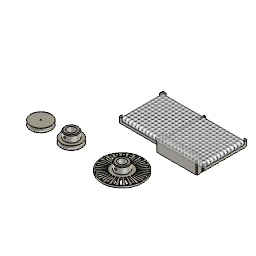
test_parts_v1 (Autodesk Fusion 360 design; units mm, degrees)
Autodesk Fusion 360 part; units mm, degrees
sketch "スケッチ1" plane through (0, 0, 0) normal (0, 0, 1) x (1, 0, 0)
  circle A0 centre (0, 0) radius 30
  circle A1 centre (0, 0) radius 6
  circle A2 centre (0, 0) radius 28.5
  circle A3 centre (0, 0) radius 10
  line L0 (0, -10) -> (0, -28.5)
  line L1 (1.3053, -9.9144) -> (3.72, -28.2562)
  line L2 (2.5882, -9.6593) -> (7.3763, -27.5289)
  line L3 (3.8268, -9.2388) -> (10.9065, -26.3306)
  line L4 (5, -8.6603) -> (14.25, -24.6817)
  line L5 (6.0876, -7.9335) -> (17.3497, -22.6106)
  line L6 (7.0711, -7.0711) -> (20.1525, -20.1525)
  line L7 (7.9335, -6.0876) -> (22.6106, -17.3497)
  line L8 (8.6603, -5) -> (24.6817, -14.25)
  line L9 (9.2388, -3.8268) -> (26.3306, -10.9065)
  line L10 (9.6593, -2.5882) -> (27.5289, -7.3763)
  line L11 (9.9144, -1.3053) -> (28.2562, -3.72)
  line L12 (10, 0) -> (28.5, 0)
  line L13 (9.9144, 1.3053) -> (28.2562, 3.72)
  line L14 (9.6593, 2.5882) -> (27.5289, 7.3763)
  line L15 (9.2388, 3.8268) -> (26.3306, 10.9065)
  line L16 (8.6603, 5) -> (24.6817, 14.25)
  line L17 (7.9335, 6.0876) -> (22.6106, 17.3497)
  line L18 (7.0711, 7.0711) -> (20.1525, 20.1525)
  line L19 (6.0876, 7.9335) -> (17.3497, 22.6106)
  line L20 (5, 8.6603) -> (14.25, 24.6817)
  line L21 (3.8268, 9.2388) -> (10.9065, 26.3306)
  line L22 (2.5882, 9.6593) -> (7.3763, 27.5289)
  line L23 (1.3053, 9.9144) -> (3.72, 28.2562)
  line L24 (0, 10) -> (0, 28.5)
  line L25 (-1.3053, 9.9144) -> (-3.72, 28.2562)
  line L26 (-2.5882, 9.6593) -> (-7.3763, 27.5289)
  line L27 (-3.8268, 9.2388) -> (-10.9065, 26.3306)
  line L28 (-5, 8.6603) -> (-14.25, 24.6817)
  line L29 (-6.0876, 7.9335) -> (-17.3497, 22.6106)
  line L30 (-7.0711, 7.0711) -> (-20.1525, 20.1525)
  line L31 (-7.9335, 6.0876) -> (-22.6106, 17.3497)
  line L32 (-8.6603, 5) -> (-24.6817, 14.25)
  line L33 (-9.2388, 3.8268) -> (-26.3306, 10.9065)
  line L34 (-9.6593, 2.5882) -> (-27.5289, 7.3763)
  line L35 (-9.9144, 1.3053) -> (-28.2562, 3.72)
  line L36 (-10, 0) -> (-28.5, 0)
  line L37 (-9.9144, -1.3053) -> (-28.2562, -3.72)
  line L38 (-9.6593, -2.5882) -> (-27.5289, -7.3763)
  line L39 (-9.2388, -3.8268) -> (-26.3306, -10.9065)
  line L40 (-8.6603, -5) -> (-24.6817, -14.25)
  line L41 (-7.9335, -6.0876) -> (-22.6106, -17.3497)
  line L42 (-7.0711, -7.0711) -> (-20.1525, -20.1525)
  line L43 (-6.0876, -7.9335) -> (-17.3497, -22.6106)
  line L44 (-5, -8.6603) -> (-14.25, -24.6817)
  line L45 (-3.8268, -9.2388) -> (-10.9065, -26.3306)
  line L46 (-2.5882, -9.6593) -> (-7.3763, -27.5289)
  line L47 (-1.3053, -9.9144) -> (-3.72, -28.2562)
  dimension "d1" = 60
  dimension "d2" = 12
  dimension "d3" = 57
  dimension "d5" = 360
  constraint coincident A0.centre A1.centre
  constraint concentric A0 A2
  constraint concentric A2 A3
  constraint coincident A2 L0.end
  constraint coincident A3 L0.start
  measures "d1" diameter of A0
  measures "d2" diameter of A1
  measures "d3" diameter of A2
extrude "押し出し1" add sketch "スケッチ1" along normal blind 3 contours A0 | A2 A3 L12 L13 | A2 A3 L10 L11 | A3 | A2 A3 L14 L15 | A2 A3 L8 L9 | A2 A3 L16 L17 | A2 A3 L6 L7 | A2 A3 L18 L19 | A2 A3 L4 L5 | A2 A3 L20 L21 | A2 A3 L2 L3 | A2 A3 L22 L23 | A2 A3 L0 L1 | A2 A3 L24 L25 | A2 A3 L46 L47 | A2 A3 L26 L27 | A2 A3 L44 L45 | A2 A3 L28 L29 | A2 A3 L42 L43 | A2 A3 L30 L31 | A2 A3 L40 L41 | A2 A3 L32 L33 | A2 A3 L38 L39 | A2 A3 L34 L35 | A2 A3 L36 L37 makes body 1
sketch "スケッチ2" plane through (0, 0, 0) normal (0, 0, 1) x (1, 0, 0)
  circle A0 centre (0, 0) radius 15
  circle A1 centre (0, 0) radius 6
  circle A2 centre (0, 0) radius 6
  constraint coincident A0.centre A1.centre
  constraint concentric A0 A2
extrude "押し出し2" add sketch "スケッチ2" along normal blind 3 bodies 1
sketch "スケッチ3" plane through (0, 0, 3) normal (0, 0, 1) x (-1, 0, 0)
  line L0 (3.8823, -14.4889) -> (7.3763, -27.5289)
  arc A0 (3.72, -28.2562) -> (7.3763, -27.5289) centre (0, 0) ccw
  line L1 (3.72, -28.2562) -> (1.9579, -14.8717)
  arc A1 (1.9579, -14.8717) -> (3.8823, -14.4889) centre (0, 0) ccw
  arc A2 (5.7403, -13.8582) -> (7.5, -12.9904) centre (0, 0) ccw
  line L2 (7.5, -12.9904) -> (14.25, -24.6817)
  arc A3 (10.9065, -26.3306) -> (14.25, -24.6817) centre (0, 0) ccw
  line L3 (10.9065, -26.3306) -> (5.7403, -13.8582)
  line L4 (0, -15) -> (0, -28.5)
  arc A4 (-3.72, -28.2562) -> (0, -28.5) centre (0, 0) ccw
  line L5 (-3.72, -28.2562) -> (-1.9579, -14.8717)
  arc A5 (-1.9579, -14.8717) -> (0, -15) centre (0, 0) ccw
  arc A6 (9.1314, -11.9003) -> (10.6066, -10.6066) centre (0, 0) ccw
  line L6 (10.6066, -10.6066) -> (20.1525, -20.1525)
  arc A7 (17.3497, -22.6106) -> (20.1525, -20.1525) centre (0, 0) ccw
  line L7 (17.3497, -22.6106) -> (9.1314, -11.9003)
  line L8 (-3.8823, -14.4889) -> (-7.3763, -27.5289)
  arc A8 (-10.9065, -26.3306) -> (-7.3763, -27.5289) centre (0, 0) ccw
  line L9 (-10.9065, -26.3306) -> (-5.7403, -13.8582)
  arc A9 (-5.7403, -13.8582) -> (-3.8823, -14.4889) centre (0, 0) ccw
  arc A10 (11.9003, -9.1314) -> (12.9904, -7.5) centre (0, 0) ccw
  line L10 (12.9904, -7.5) -> (24.6817, -14.25)
  arc A11 (22.6106, -17.3497) -> (24.6817, -14.25) centre (0, 0) ccw
  line L11 (22.6106, -17.3497) -> (11.9003, -9.1314)
  line L12 (-7.5, -12.9904) -> (-14.25, -24.6817)
  arc A12 (-17.3497, -22.6106) -> (-14.25, -24.6817) centre (0, 0) ccw
  line L13 (-17.3497, -22.6106) -> (-9.1314, -11.9003)
  arc A13 (-9.1314, -11.9003) -> (-7.5, -12.9904) centre (0, 0) ccw
  arc A14 (13.8582, -5.7403) -> (14.4889, -3.8823) centre (0, 0) ccw
  line L14 (14.4889, -3.8823) -> (27.5289, -7.3763)
  arc A15 (26.3306, -10.9065) -> (27.5289, -7.3763) centre (0, 0) ccw
  line L15 (26.3306, -10.9065) -> (13.8582, -5.7403)
  line L16 (-10.6066, -10.6066) -> (-20.1525, -20.1525)
  arc A16 (-22.6106, -17.3497) -> (-20.1525, -20.1525) centre (0, 0) ccw
  line L17 (-22.6106, -17.3497) -> (-11.9003, -9.1314)
  arc A17 (-11.9003, -9.1314) -> (-10.6066, -10.6066) centre (0, 0) ccw
  arc A18 (14.8717, -1.9579) -> (15, 0) centre (0, 0) ccw
  line L18 (15, 0) -> (28.5, 0)
  arc A19 (28.2562, -3.72) -> (28.5, 0) centre (0, 0) ccw
  line L19 (28.2562, -3.72) -> (14.8717, -1.9579)
  line L20 (-12.9904, -7.5) -> (-24.6817, -14.25)
  arc A20 (-26.3306, -10.9065) -> (-24.6817, -14.25) centre (0, 0) ccw
  line L21 (-26.3306, -10.9065) -> (-13.8582, -5.7403)
  arc A21 (-13.8582, -5.7403) -> (-12.9904, -7.5) centre (0, 0) ccw
  arc A22 (14.8717, 1.9579) -> (14.4889, 3.8823) centre (0, 0) ccw
  line L22 (14.4889, 3.8823) -> (27.5289, 7.3763)
  arc A23 (28.2562, 3.72) -> (27.5289, 7.3763) centre (0, 0) ccw
  line L23 (28.2562, 3.72) -> (14.8717, 1.9579)
  line L24 (-14.4889, -3.8823) -> (-27.5289, -7.3763)
  arc A24 (-28.2562, -3.72) -> (-27.5289, -7.3763) centre (0, 0) ccw
  line L25 (-28.2562, -3.72) -> (-14.8717, -1.9579)
  arc A25 (-14.8717, -1.9579) -> (-14.4889, -3.8823) centre (0, 0) ccw
  arc A26 (13.8582, 5.7403) -> (12.9904, 7.5) centre (0, 0) ccw
  line L26 (12.9904, 7.5) -> (24.6817, 14.25)
  arc A27 (26.3306, 10.9065) -> (24.6817, 14.25) centre (0, 0) ccw
  line L27 (26.3306, 10.9065) -> (13.8582, 5.7403)
  line L28 (-15, 0) -> (-28.5, 0)
  arc A28 (-28.2562, 3.72) -> (-28.5, 0) centre (0, 0) ccw
  line L29 (-28.2562, 3.72) -> (-14.8717, 1.9579)
  arc A29 (-14.8717, 1.9579) -> (-15, 0) centre (0, 0) ccw
  arc A30 (11.9003, 9.1314) -> (10.6066, 10.6066) centre (0, 0) ccw
  line L30 (10.6066, 10.6066) -> (20.1525, 20.1525)
  arc A31 (22.6106, 17.3497) -> (20.1525, 20.1525) centre (0, 0) ccw
  line L31 (22.6106, 17.3497) -> (11.9003, 9.1314)
  line L32 (-14.4889, 3.8823) -> (-27.5289, 7.3763)
  arc A32 (-26.3306, 10.9065) -> (-27.5289, 7.3763) centre (0, 0) ccw
  line L33 (-26.3306, 10.9065) -> (-13.8582, 5.7403)
  arc A33 (-13.8582, 5.7403) -> (-14.4889, 3.8823) centre (0, 0) ccw
  arc A34 (9.1314, 11.9003) -> (7.5, 12.9904) centre (0, 0) ccw
  line L34 (7.5, 12.9904) -> (14.25, 24.6817)
  arc A35 (17.3497, 22.6106) -> (14.25, 24.6817) centre (0, 0) ccw
  line L35 (17.3497, 22.6106) -> (9.1314, 11.9003)
  line L36 (-12.9904, 7.5) -> (-24.6817, 14.25)
  arc A36 (-22.6106, 17.3497) -> (-24.6817, 14.25) centre (0, 0) ccw
  line L37 (-22.6106, 17.3497) -> (-11.9003, 9.1314)
  arc A37 (-11.9003, 9.1314) -> (-12.9904, 7.5) centre (0, 0) ccw
  arc A38 (5.7403, 13.8582) -> (3.8823, 14.4889) centre (0, 0) ccw
  line L38 (3.8823, 14.4889) -> (7.3763, 27.5289)
  arc A39 (10.9065, 26.3306) -> (7.3763, 27.5289) centre (0, 0) ccw
  line L39 (10.9065, 26.3306) -> (5.7403, 13.8582)
  line L40 (-10.6066, 10.6066) -> (-20.1525, 20.1525)
  arc A40 (-17.3497, 22.6106) -> (-20.1525, 20.1525) centre (0, 0) ccw
  line L41 (-17.3497, 22.6106) -> (-9.1314, 11.9003)
  arc A41 (-9.1314, 11.9003) -> (-10.6066, 10.6066) centre (0, 0) ccw
  arc A42 (1.9579, 14.8717) -> (0, 15) centre (0, 0) ccw
  line L42 (0, 15) -> (0, 28.5)
  arc A43 (3.72, 28.2562) -> (0, 28.5) centre (0, 0) ccw
  line L43 (3.72, 28.2562) -> (1.9579, 14.8717)
  line L44 (-7.5, 12.9904) -> (-14.25, 24.6817)
  arc A44 (-10.9065, 26.3306) -> (-14.25, 24.6817) centre (0, 0) ccw
  line L45 (-10.9065, 26.3306) -> (-5.7403, 13.8582)
  arc A45 (-5.7403, 13.8582) -> (-7.5, 12.9904) centre (0, 0) ccw
  circle A46 centre (0, 0) radius 6
  circle A47 centre (0, 0) radius 30
  arc A48 (-1.9579, 14.8717) -> (-3.8823, 14.4889) centre (0, 0) ccw
  line L46 (-3.8823, 14.4889) -> (-7.3763, 27.5289)
  arc A49 (-3.72, 28.2562) -> (-7.3763, 27.5289) centre (0, 0) ccw
  line L47 (-3.72, 28.2562) -> (-1.9579, 14.8717)
  circle A50 centre (0, 0) radius 10
  constraint concentric A0 A50
extrude "押し出し3" add sketch "スケッチ3" along normal blind 10 contours A50 bodies 1
chamfer "面取り1" distance 1 angle 45 1 edges at (9.3233, 3.6162, 13) on bodies 1
sketch "スケッチ4" plane through (0, 0, 0) normal (1, 0, 0) x (0, 1, 0)
  line L0 (0, 3) -> (0, 6)
  constraint vertical L0
sketch "スケッチ5" plane through (0, 0, 0) normal (0, 0, 1) x (1, 0, 0)
sketch "スケッチ6" plane through (0, 0, 0) normal (0, 0, 1) x (1, 0, 0)
  circle A0 centre (-75, 0) radius 15
  circle A1 centre (-75, 0) radius 6
  dimension "d16" = 12
  constraint concentric A0 A1
  measures "d16" diameter of A1
extrude "押し出し4" add sketch "スケッチ6" along normal blind 6 separate body makes body 2
sketch "スケッチ7" plane through (0, 0, 6) normal (0, 0, 1) x (-1, 0, 0)
  circle A0 centre (75, 0) radius 6
  circle A1 centre (75, 0) radius 15
  circle A2 centre (75, 0) radius 10
  constraint concentric A0 A2
extrude "押し出し5" add sketch "スケッチ7" along normal blind 10 contours A2 bodies 2
sketch "スケッチ8" plane through (0, 0, 0) normal (0, 1, 0) x (1, 0, 0)
  circle A0 centre (-90, -3) radius 2.75
  line L0 (-75, 0) -> (-75, -16)
  dimension "d21" = 5.5
  constraint vertical L0
  measures "d21" diameter of A0
revolve "回転1" cut sketch "スケッチ8" angle 360 about axis through (-75, 0, 0) along (0, 0, 1) bodies 2
chamfer "面取り2" distance 1 angle 45 1 edges at (-65.6767, 3.6162, 16) on bodies 2
sketch "スケッチ9" plane through (0, 0, 0) normal (0, 0, 1) x (1, 0, 0)
  circle A0 centre (-120, 0) radius 15
  circle A1 centre (-120, 0) radius 0.9
  dimension "d25" = 1.8
  constraint concentric A0 A1
  measures "d25" diameter of A1
extrude "押し出し6" add sketch "スケッチ9" along normal blind 6 separate body makes body 3
sketch "スケッチ10" plane through (0, 0, 0) normal (0, 1, 0) x (1, 0, 0)
  line L0 (-120, 0) -> (-120, -10)
  circle A0 centre (-135, -3) radius 2.75
  dimension "d28" = 5.5
  constraint vertical L0
  measures "d28" diameter of A0
revolve "回転2" cut sketch "スケッチ10" angle 360 about axis through (-120, 0, 0) along (0, 0, 1) bodies 3
sketch "スケッチ11" plane through (0, 0, 0) normal (0, 0, 1) x (1, 0, 0)
  line L0 (0, 50) -> (60, 50)
  line L1 (60, 50) -> (60, 59)
  line L2 (60, 59) -> (0, 59)
  line L3 (0, 59) -> (0, 50)
  dimension "d30" = 60
  dimension "d31" = 9
  constraint horizontal L0
  constraint vertical L1
  constraint horizontal L2
  constraint vertical L3
  measures "d30" distance of L0.start L0.end
  measures "d31" distance of L0.start L2.end
extrude "押し出し7" add sketch "スケッチ11" along normal blind 18 separate body makes body 4
sketch "スケッチ12" plane through (0, 0, 18) normal (0, 0, 1) x (-1, 0, 0)
  line L0 (0, -59) -> (0, -50)
  line L1 (0, -50) -> (-60, -50)
  line L2 (-60, -50) -> (-60, -59)
  line L3 (-60, -59) -> (0, -59)
  line L4 (0, -54.5) -> (-60, -54.5)
  line L5 (-60, -54.5) -> (-54.5, -54.5)
  line L6 (0, -54.5) -> (-5.5, -54.5)
  circle A0 centre (-5.5, -54.5) radius 2
  circle A1 centre (-54.5, -54.5) radius 2
  dimension "d34" = 5.5
  dimension "d35" = 5.5
  dimension "d36" = 4
  dimension "d37" = 4
  constraint midpoint L0 L4.start
  constraint midpoint L2 L4.end
  constraint perpendicular L2 L5
  constraint perpendicular L0 L6
  constraint coincident L6.end A0.centre
  constraint coincident L5.end A1.centre
  measures "d34" distance of L4.end L5.end
  measures "d35" distance of L4.start L6.end
  measures "d36" diameter of A0
  measures "d37" diameter of A1
extrude "押し出し8" add sketch "スケッチ12" along normal blind 7 contours L4 L6 A0 | L4 L6 A0 | L4 L5 A1 | L4 L5 A1 bodies 4
chamfer "面取り3" distance 1 angle 45 2 faces at (6.394, 54.1665, 25) (55.4926, 54.1814, 25) on bodies 4
chamfer "面取り4" distance 1 angle 45 4 edges at (60, 50, 9) (60, 59, 9) (0, 50, 9) (0, 59, 9) on bodies 4
sketch "スケッチ13" plane through (0, 0, 0) normal (0, 0, -1) x (1, 0, 0)
  line L0 (0, -58) -> (1, -59)
  line L1 (1, -59) -> (59, -59)
  line L2 (59, -59) -> (60, -58)
  line L3 (60, -58) -> (60, -51)
  line L4 (60, -51) -> (59, -50)
  line L5 (59, -50) -> (1, -50)
  line L6 (1, -50) -> (0, -51)
  line L7 (0, -51) -> (0, -58)
  line L8 (0, -54.5) -> (60, -54.5)
  line L9 (0, -54.5) -> (5, -54.5)
  line L10 (60, -54.5) -> (55, -54.5)
  constraint midpoint L7 L8.start
  constraint midpoint L3 L8.end
  constraint coincident L8 L9.end
  constraint coincident L8 L10.end
hole "穴2" at (5, 54.5, 0) at (55, 54.5, 0) direction (0, 0, 1) diameter 2.9 depth 5 tip angle 180 bodies 4
sketch "スケッチ14" plane through (0, 0, 0) normal (0, 0, 1) x (1, 0, 0)
  line L0 (60, 60) -> (-65, 60)
  line L1 (-65, 60) -> (-65, 125)
  line L2 (-65, 125) -> (60, 125)
  line L3 (60, 125) -> (60, 60)
  dimension "d45" = 125
  dimension "d46" = 65
  constraint horizontal L0
  constraint vertical L1
  constraint horizontal L2
  constraint vertical L3
  measures "d45" distance of L0.start L0.end
  measures "d46" distance of L0.start L2.end
sketch "スケッチ15" plane through (0, 0, 0) normal (0, 0, 1) x (1, 0, 0)
extrude "押し出し9" add sketch "スケッチ14" along normal blind 4 separate body makes body 5
sketch "スケッチ16" plane through (0, 0, 4) normal (0, 0, 1) x (-1, 0, 0)
  line L0 (-60, -125) -> (65, -125)
  line L1 (65, -125) -> (65, -60)
  line L2 (65, -60) -> (-60, -60)
  line L3 (-60, -60) -> (-60, -125)
sketch "スケッチ17" plane through (0, 0, 4) normal (0, 0, 1) x (-1, 0, 0)
  point P0 (60, -120)
  point P1 (60, -115)
  point P2 (60, -110)
  point P3 (60, -105)
  point P4 (60, -100)
  point P5 (60, -95)
  point P6 (60, -90)
  point P7 (60, -85)
  point P8 (60, -80)
  point P9 (60, -75)
  point P10 (60, -70)
  point P11 (60, -65)
  point P12 (55, -120)
  point P13 (55, -115)
  point P14 (55, -110)
  point P15 (55, -105)
  point P16 (55, -100)
  point P17 (55, -95)
  point P18 (55, -90)
  point P19 (55, -85)
  point P20 (55, -80)
  point P21 (55, -75)
  point P22 (55, -70)
  point P23 (55, -65)
  point P24 (50, -120)
  point P25 (50, -115)
  point P26 (50, -110)
  point P27 (50, -105)
  point P28 (50, -100)
  point P29 (50, -95)
  point P30 (50, -90)
  point P31 (50, -85)
  point P32 (50, -80)
  point P33 (50, -75)
  point P34 (50, -70)
  point P35 (50, -65)
  point P36 (45, -120)
  point P37 (45, -115)
  point P38 (45, -110)
  point P39 (45, -105)
  point P40 (45, -100)
  point P41 (45, -95)
  point P42 (45, -90)
  point P43 (45, -85)
  point P44 (45, -80)
  point P45 (45, -75)
  point P46 (45, -70)
  point P47 (45, -65)
  point P48 (40, -120)
  point P49 (40, -115)
  point P50 (40, -110)
  point P51 (40, -105)
  point P52 (40, -100)
  point P53 (40, -95)
  point P54 (40, -90)
  point P55 (40, -85)
  point P56 (40, -80)
  point P57 (40, -75)
  point P58 (40, -70)
  point P59 (40, -65)
  point P60 (35, -120)
  point P61 (35, -115)
  point P62 (35, -110)
  point P63 (35, -105)
  point P64 (35, -100)
  point P65 (35, -95)
  point P66 (35, -90)
  point P67 (35, -85)
  point P68 (35, -80)
  point P69 (35, -75)
  point P70 (35, -70)
  point P71 (35, -65)
  point P72 (30, -120)
  point P73 (30, -115)
  point P74 (30, -110)
  point P75 (30, -105)
  point P76 (30, -100)
  point P77 (30, -95)
  point P78 (30, -90)
  point P79 (30, -85)
  point P80 (30, -80)
  point P81 (30, -75)
  point P82 (30, -70)
  point P83 (30, -65)
  point P84 (25, -120)
  point P85 (25, -115)
  point P86 (25, -110)
  point P87 (25, -105)
  point P88 (25, -100)
  point P89 (25, -95)
  point P90 (25, -90)
  point P91 (25, -85)
  point P92 (25, -80)
  point P93 (25, -75)
  point P94 (25, -70)
  point P95 (25, -65)
  point P96 (20, -120)
  point P97 (20, -115)
  point P98 (20, -110)
  point P99 (20, -105)
  point P100 (20, -100)
  point P101 (20, -95)
  point P102 (20, -90)
  point P103 (20, -85)
  point P104 (20, -80)
  point P105 (20, -75)
  point P106 (20, -70)
  point P107 (20, -65)
  point P108 (15, -120)
  point P109 (15, -115)
  point P110 (15, -110)
  point P111 (15, -105)
  point P112 (15, -100)
  point P113 (15, -95)
  point P114 (15, -90)
  point P115 (15, -85)
  point P116 (15, -80)
  point P117 (15, -75)
  point P118 (15, -70)
  point P119 (15, -65)
  point P120 (10, -120)
  point P121 (10, -115)
  point P122 (10, -110)
  point P123 (10, -105)
  point P124 (10, -100)
  point P125 (10, -95)
  point P126 (10, -90)
  point P127 (10, -85)
  point P128 (10, -80)
  point P129 (10, -75)
  point P130 (10, -70)
  point P131 (10, -65)
  point P132 (5, -120)
  point P133 (5, -115)
  point P134 (5, -110)
  point P135 (5, -105)
  point P136 (5, -100)
  point P137 (5, -95)
  point P138 (5, -90)
  point P139 (5, -85)
  point P140 (5, -80)
  point P141 (5, -75)
  point P142 (5, -70)
  point P143 (5, -65)
  point P144 (0, -120)
  point P145 (0, -115)
  point P146 (0, -110)
  point P147 (0, -105)
  point P148 (0, -100)
  point P149 (0, -95)
  point P150 (0, -90)
  point P151 (0, -85)
  point P152 (0, -80)
  point P153 (0, -75)
  point P154 (0, -70)
  point P155 (0, -65)
  point P156 (-5, -120)
  point P157 (-5, -115)
  point P158 (-5, -110)
  point P159 (-5, -105)
  point P160 (-5, -100)
  point P161 (-5, -95)
  point P162 (-5, -90)
  point P163 (-5, -85)
  point P164 (-5, -80)
  point P165 (-5, -75)
  point P166 (-5, -70)
  point P167 (-5, -65)
  point P168 (-10, -120)
  point P169 (-10, -115)
  point P170 (-10, -110)
  point P171 (-10, -105)
  point P172 (-10, -100)
  point P173 (-10, -95)
  point P174 (-10, -90)
  point P175 (-10, -85)
  point P176 (-10, -80)
  point P177 (-10, -75)
  point P178 (-10, -70)
  point P179 (-10, -65)
  point P180 (-15, -120)
  point P181 (-15, -115)
  point P182 (-15, -110)
  point P183 (-15, -105)
  point P184 (-15, -100)
  point P185 (-15, -95)
  point P186 (-15, -90)
  point P187 (-15, -85)
  point P188 (-15, -80)
  point P189 (-15, -75)
  point P190 (-15, -70)
  point P191 (-15, -65)
  point P192 (-20, -120)
  point P193 (-20, -115)
  point P194 (-20, -110)
  point P195 (-20, -105)
  point P196 (-20, -100)
  point P197 (-20, -95)
  point P198 (-20, -90)
  point P199 (-20, -85)
  point P200 (-20, -80)
  point P201 (-20, -75)
  point P202 (-20, -70)
  point P203 (-20, -65)
  point P204 (-25, -120)
  point P205 (-25, -115)
  point P206 (-25, -110)
  point P207 (-25, -105)
  point P208 (-25, -100)
  point P209 (-25, -95)
  point P210 (-25, -90)
  point P211 (-25, -85)
  point P212 (-25, -80)
  point P213 (-25, -75)
  point P214 (-25, -70)
  point P215 (-25, -65)
  point P216 (-30, -120)
  point P217 (-30, -115)
  point P218 (-30, -110)
  point P219 (-30, -105)
  point P220 (-30, -100)
  point P221 (-30, -95)
  point P222 (-30, -90)
  point P223 (-30, -85)
  point P224 (-30, -80)
  point P225 (-30, -75)
  point P226 (-30, -70)
  point P227 (-30, -65)
  point P228 (-35, -120)
  point P229 (-35, -115)
  point P230 (-35, -110)
  point P231 (-35, -105)
  point P232 (-35, -100)
  point P233 (-35, -95)
  point P234 (-35, -90)
  point P235 (-35, -85)
  point P236 (-35, -80)
  point P237 (-35, -75)
  point P238 (-35, -70)
  point P239 (-35, -65)
  point P240 (-40, -120)
  point P241 (-40, -115)
  point P242 (-40, -110)
  point P243 (-40, -105)
  point P244 (-40, -100)
  point P245 (-40, -95)
  point P246 (-40, -90)
  point P247 (-40, -85)
  point P248 (-40, -80)
  point P249 (-40, -75)
  point P250 (-40, -70)
  point P251 (-40, -65)
  point P252 (-45, -120)
  point P253 (-45, -115)
  point P254 (-45, -110)
  point P255 (-45, -105)
  point P256 (-45, -100)
  point P257 (-45, -95)
  point P258 (-45, -90)
  point P259 (-45, -85)
  point P260 (-45, -80)
  point P261 (-45, -75)
  point P262 (-45, -70)
  point P263 (-45, -65)
  point P264 (-50, -120)
  point P265 (-50, -115)
  point P266 (-50, -110)
  point P267 (-50, -105)
  point P268 (-50, -100)
  point P269 (-50, -95)
  point P270 (-50, -90)
  point P271 (-50, -85)
  point P272 (-50, -80)
  point P273 (-50, -75)
  point P274 (-50, -70)
  point P275 (-50, -65)
  point P276 (-55, -120)
  point P277 (-55, -115)
  point P278 (-55, -110)
  point P279 (-55, -105)
  point P280 (-55, -100)
  point P281 (-55, -95)
  point P282 (-55, -90)
  point P283 (-55, -85)
  point P284 (-55, -80)
  point P285 (-55, -75)
  point P286 (-55, -70)
  point P287 (-55, -65)
  dimension "d54" = -115
  dimension "d55" = 0
hole "穴4" at (-60, 120, 4) at (-25, 90, 4) at (-25, 95, 4) at (-25, 100, 4) at (-25, 110, 4) at (-25, 120, 4) at (-60, 105, 4) at (-60, 100, 4) at (-60, 95, 4) at (-60, 90, 4) at (-60, 85, 4) at (-60, 80, 4) at (-60, 75, 4) at (-60, 70, 4) at (-60, 65, 4) at (-55, 65, 4) at (-55, 70, 4) at (-55, 75, 4) at (-55, 80, 4) at (-55, 85, 4) at (-55, 90, 4) at (-55, 95, 4) at (-55, 100, 4) at (-55, 105, 4) at (-55, 110, 4) at (-55, 115, 4) at (-55, 120, 4) at (-60, 115, 4) at (-60, 110, 4) at (-50, 120, 4) at (-50, 115, 4) at (-50, 110, 4) at (-50, 105, 4) at (-50, 100, 4) at (-50, 95, 4) at (-50, 90, 4) at (-50, 85, 4) at (-50, 80, 4) at (-50, 75, 4) at (-50, 70, 4) at (-50, 65, 4) at (-45, 65, 4) at (-45, 70, 4) at (-45, 75, 4) at (-45, 80, 4) at (-45, 85, 4) at (-45, 90, 4) at (-45, 95, 4) at (-45, 100, 4) at (-45, 105, 4) at (-45, 110, 4) at (-45, 115, 4) at (-45, 120, 4) at (-40, 120, 4) at (-40, 115, 4) at (-40, 110, 4) at (-40, 105, 4) at (-40, 100, 4) at (-40, 95, 4) at (-40, 90, 4) at (-40, 85, 4) at (-40, 80, 4) at (-40, 75, 4) at (-40, 70, 4) at (-40, 65, 4) at (-35, 65, 4) at (-35, 70, 4) at (-35, 75, 4) at (-35, 80, 4) at (-35, 85, 4) at (-35, 90, 4) at (-35, 95, 4) at (-35, 100, 4) at (-35, 105, 4) at (-35, 110, 4) at (-35, 115, 4) at (-35, 120, 4) at (-30, 120, 4) at (-30, 115, 4) at (-30, 110, 4) at (-30, 100, 4) at (-30, 95, 4) at (-30, 90, 4) at (-30, 85, 4) at (-30, 75, 4) at (-30, 70, 4) at (-30, 65, 4) at (-25, 65, 4) at (-25, 70, 4) at (-25, 85, 4) at (-20, 65, 4) at (-20, 70, 4) at (-15, 85, 4) at (-15, 90, 4) at (-15, 95, 4) at (-15, 100, 4) at (-15, 105, 4) at (-20, 115, 4) at (-20, 120, 4) at (-20, 110, 4) at (-20, 105, 4) at (-20, 85, 4) at (-20, 80, 4) at (-20, 75, 4) at (-20, 90, 4) at (-20, 95, 4) at (-20, 100, 4) at (-15, 120, 4) at (-10, 120, 4) at (-5, 115, 4) at (0, 115, 4) at (5, 115, 4) at (10, 115, 4) at (25, 115, 4) at (5, 120, 4) at (0, 120, 4) at (-5, 120, 4) at (-15, 115, 4) at (-15, 110, 4) at (-10, 110, 4) at (0, 110, 4) at (15, 105, 4) at (20, 105, 4) at (25, 105, 4) at (10, 105, 4) at (5, 105, 4) at (0, 105, 4) at (-10, 105, 4) at (25, 100, 4) at (30, 100, 4) at (20, 100, 4) at (-10, 95, 4) at (-10, 90, 4) at (-5, 90, 4) at (5, 90, 4) at (10, 90, 4) at (15, 90, 4) at (0, 90, 4) at (20, 85, 4) at (25, 85, 4) at (10, 85, 4) at (5, 85, 4) at (0, 85, 4) at (-5, 85, 4) at (15, 80, 4) at (20, 80, 4) at (25, 80, 4) at (10, 80, 4) at (5, 80, 4) at (25, 75, 4) at (30, 75, 4) at (35, 75, 4) at (40, 75, 4) at (-5, 80, 4) at (-10, 80, 4) at (-15, 80, 4) at (-15, 75, 4) at (-10, 75, 4) at (-5, 75, 4) at (0, 75, 4) at (5, 75, 4) at (10, 70, 4) at (15, 70, 4) at (20, 70, 4) at (25, 70, 4) at (30, 65, 4) at (35, 65, 4) at (40, 65, 4) at (45, 65, 4) at (25, 65, 4) at (20, 65, 4) at (15, 65, 4) at (10, 65, 4) at (5, 65, 4) at (0, 65, 4) at (-5, 65, 4) at (-10, 65, 4) at (-15, 65, 4) at (-15, 70, 4) at (-10, 70, 4) at (-5, 70, 4) at (0, 70, 4) at (5, 70, 4) at (30, 70, 4) at (35, 70, 4) at (40, 70, 4) at (45, 70, 4) at (50, 65, 4) at (50, 70, 4) at (55, 70, 4) at (55, 65, 4) at (55, 75, 4) at (55, 80, 4) at (55, 85, 4) at (55, 90, 4) at (-25, 115, 4) at (-25, 105, 4) at (-30, 105, 4) at (-30, 80, 4) at (-25, 80, 4) at (-25, 75, 4) at (-10, 85, 4) at (0, 80, 4) at (10, 75, 4) at (15, 75, 4) at (20, 75, 4) at (50, 75, 4) at (50, 80, 4) at (50, 85, 4) at (50, 90, 4) at (50, 95, 4) at (50, 100, 4) at (50, 105, 4) at (50, 110, 4) at (50, 115, 4) at (50, 120, 4) at (55, 120, 4) at (55, 115, 4) at (55, 110, 4) at (55, 105, 4) at (55, 100, 4) at (55, 95, 4) at (45, 120, 4) at (45, 115, 4) at (45, 110, 4) at (45, 105, 4) at (45, 100, 4) at (45, 95, 4) at (45, 90, 4) at (45, 85, 4) at (45, 80, 4) at (45, 75, 4) at (40, 80, 4) at (40, 85, 4) at (40, 90, 4) at (40, 95, 4) at (40, 100, 4) at (40, 105, 4) at (40, 110, 4) at (40, 115, 4) at (40, 120, 4) at (35, 120, 4) at (35, 115, 4) at (35, 110, 4) at (35, 105, 4) at (35, 100, 4) at (35, 95, 4) at (35, 90, 4) at (35, 85, 4) at (35, 80, 4) at (30, 80, 4) at (30, 85, 4) at (30, 90, 4) at (30, 95, 4) at (25, 95, 4) at (20, 95, 4) at (20, 90, 4) at (25, 90, 4) at (15, 85, 4) at (15, 95, 4) at (10, 95, 4) at (5, 95, 4) at (0, 95, 4) at (-5, 95, 4) at (-5, 100, 4) at (0, 100, 4) at (5, 100, 4) at (10, 100, 4) at (15, 100, 4) at (30, 105, 4) at (30, 110, 4) at (30, 115, 4) at (30, 120, 4) at (25, 120, 4) at (20, 120, 4) at (15, 120, 4) at (10, 120, 4) at (15, 115, 4) at (20, 115, 4) at (20, 110, 4) at (25, 110, 4) at (15, 110, 4) at (10, 110, 4) at (5, 110, 4) at (-5, 110, 4) at (-5, 105, 4) at (-10, 100, 4) at (-10, 115, 4) direction (0, 0, -1) diameter 2.9 depth 4 tip angle 180 bodies 5
sketch "スケッチ18" plane through (0, 0, 4) normal (0, 0, 1) x (-1, 0, 0)
  line L0 (-60, -125) -> (-60, -120)
  line L1 (-60, -120) -> (-55, -125)
  line L2 (-55, -125) -> (-60, -125)
  line L3 (65, -125) -> (65, -120)
  line L4 (65, -120) -> (60, -125)
  line L5 (60, -125) -> (65, -125)
  line L6 (65, -60) -> (60, -60)
  line L7 (60, -60) -> (65, -65)
  line L8 (65, -65) -> (65, -60)
  line L9 (-60, -60) -> (-60, -65)
  line L10 (-60, -65) -> (-55, -60)
  line L11 (-55, -60) -> (-60, -60)
  constraint vertical L0
  constraint perpendicular L0 L2
  constraint perpendicular L2 L3
  constraint perpendicular L3 L5
  constraint perpendicular L3 L6
  constraint perpendicular L4 L7
  constraint perpendicular L6 L8
  constraint perpendicular L6 L9
  constraint perpendicular L7 L10
  constraint perpendicular L9 L11
extrude "押し出し10" add sketch "スケッチ18" along normal blind 4 bodies 5
sketch "スケッチ19" plane through (0, 0, 4) normal (0, 0, 1) x (-1, 0, 0)
  line L0 (65, -125) -> (-60, -60)
  line L1 (-60, -60) -> (-60, -125)
  line L2 (-60, -125) -> (65, -60)
  line L3 (65, -60) -> (2.5, -60)
  line L4 (2.5, -60) -> (2.5, -125)
  line L5 (2.5, -60) -> (3.5, -60)
  line L6 (3.5, -60) -> (3.5, -125)
  line L7 (3.5, -125) -> (2.5, -125)
  line L8 (2.5, -125) -> (2.5, -60)
  line L9 (2.5, -60) -> (1.5, -60)
  line L10 (1.5, -60) -> (1.5, -125)
  line L11 (1.5, -125) -> (2.5, -125)
  line L12 (2.5, -125) -> (2.5, -60)
  dimension "d61" = 1
  dimension "d62" = 1
  constraint vertical L1
  constraint horizontal L3
  constraint perpendicular L3 L4
  constraint horizontal L5
  constraint vertical L6
  constraint horizontal L7
  constraint vertical L8
  constraint horizontal L9
  constraint vertical L10
  constraint horizontal L11
  constraint vertical L12
  measures "d61" distance of L3.end L5.end
  measures "d62" distance of L3.end L9.end
extrude "押し出し11" add sketch "スケッチ19" along normal blind 4 contours L0 L4 L6 L7 L8 L12 | L0 L2 L6 | L0 L2 L10 | L2 L4 L8 L10 L11 L12 | L2 L3 L4 L5 L6 L8 L12 | L0 L4 L8 L9 L10 L12 bodies 5
chamfer "面取り5" distance 1 angle 45 4 edges at (60, 125, 4) (-65, 125, 4) (-65, 60, 4) (60, 60, 4) on bodies 5
sketch "スケッチ20" plane through (0, 0, 0) normal (0, 1, 0) x (1, 0, 0)
  line L0 (0, -13) -> (0, -8)
  line L1 (-75, -16) -> (-75, -11)
  constraint vertical L0
  constraint vertical L1
hole "穴5" at (0, 0, 8) at (-75, 0, 11) direction (0, -1, 0) diameter 2.9 depth 11 tip angle 180 bodies 1 2
